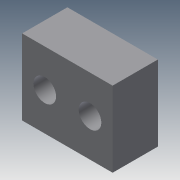
# Autodesk Inventor part: kolejnicka_ruka_druha_cast
Saved by Autodesk Inventor 2015 (Build 190159000, 159)
## iProperties
Created: 2013-03-23
Part Number: kolejnicka_ruka_druha_cast
Material: Generic
Document SubType Name: Modeling
Designer: idle-rug
Density: 1 g/cm^3
Appearance: Default
Author: idle-rug
Autodesk Inventor part; units mm, degrees
ref_plane "YZ Plane" through (0, 0, 0) normal (1, 0, 0) x (0, 1, 0)
ref_plane "XZ Plane" through (0, 0, 0) normal (0, 1, 0) x (-1, 0, 0)
ref_plane "XY Plane" through (0, 0, 0) normal (0, 0, 1) x (1, 0, 0)
sketch "Sketch1" plane through (0, 0, 0) normal (0, 1, 0) x (-1, 0, 0)
  line L0 (6, 5) -> (-6, 5)
  line L1 (-6, 5) -> (-6, -5)
  line L2 (-6, -5) -> (6, -5)
  line L3 (6, -5) -> (6, 5)
  line L4 (6, 5) -> (-6, -5) construction
  line L5 (-6, 5) -> (6, -5) construction
  point P0 (0, 0)
  dimension "d0" = 12
  dimension "d1" = 10
  constraints: 12 end point, 2 midpoint, 2 parallel, 1 horizontal, 1 perpendicular
  measures "d0" distance of L2.end L1.end
  measures "d1" distance of L1.end L0.end
extrude "Extrusion1" add sketch "Sketch1" along normal blind 6
sketch "Sketch2" plane through (0, 6, 0) normal (0, 1, 0) x (1, 0, 0)
  line L0 (6, -5) -> (6, 5) projected
  line L1 (-6, 5) -> (-6, -5) projected
  line L2 (-6, 0) -> (-3, 0)
  line L3 (6, 0) -> (3, 0)
  circle A0 centre (-3, 0) radius 1.5
  circle A1 centre (3, 0) radius 1.5
  point P0 (0, 0)
  dimension "d4" = 3
  dimension "d5" = 3
  dimension "d6" = 3
  dimension "d7" = 3
  constraints: 4 end point, 2 centre point, 2 coincident, 2 midpoint, 1 collinear, 1 perpendicular
  measures "d4" distance of L2.start L2.end
  measures "d5" distance of L3.start L3.end
  measures "d6" diameter of A0
  measures "d7" diameter of A1
extrude "Extrusion2" cut sketch "Sketch2" against normal blind 6
sketch "Sketch3" plane through (0, 0, 0) normal (0, -1, 0) x (1, 0, 0)
  circle A0 centre (-3, 0) radius 1.5 projected
  circle A1 centre (3, 0) radius 1.5 projected
  point P0 (0, 0)
extrude "Extrusion3" add sketch "Sketch3" against normal blind 6
sketch "Sketch4" plane through (0, 0, 0) normal (0, -1, 0) x (1, 0, 0)
  line L0 (-6, -5) -> (-6, 5) projected
  line L1 (6, 5) -> (6, -5) projected
  line L2 (-6, 0) -> (-3, 0)
  line L3 (-3, 0) -> (3, 0)
  circle A0 centre (3, 0) radius 1.5
  circle A1 centre (-3, 0) radius 1.5
  point P0 (0, 0)
  dimension "d12" = 3
  dimension "d13" = 6
  dimension "d14" = 3
  dimension "d15" = 3
  constraints: 4 end point, 2 centre point, 2 coincident, 1 collinear, 1 midpoint, 1 perpendicular
  measures "d12" distance of L2.start L2.end
  measures "d13" distance of L2.end L3.end
  measures "d14" diameter of A0
  measures "d15" diameter of A1
extrude "Extrusion4" cut sketch "Sketch4" against normal blind 6
body "Solid1"
